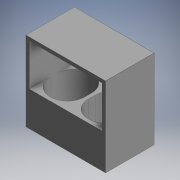
# Autodesk Inventor part: Manifold0
Saved by Autodesk Inventor 2018 (Build 220112000, 112)
## iProperties
Created: 2018-09-29
Part Number: Manifold0
Material: Generic
Document SubType Name: Modeling
Designer: Isaac Newcomb
Density: 1 g/cm^3
Appearance: Default
Author: Isaac Newcomb
Autodesk Inventor part; units mm, degrees
ref_plane "YZ Plane" through (0, 0, 0) normal (1, 0, 0) x (0, 1, 0)
ref_plane "XZ Plane" through (0, 0, 0) normal (0, 1, 0) x (-1, 0, 0)
ref_plane "XY Plane" through (0, 0, 0) normal (0, 0, 1) x (1, 0, 0)
sketch "Base Sketch" plane through (0, 0, 0) normal (0, 0, 1) x (1, 0, 0)
  line L0 (-10.5, -6) -> (10.5, -6)
  line L1 (10.5, -6) -> (10.5, 6)
  line L2 (10.5, 6) -> (-10.5, 6)
  line L3 (-10.5, 6) -> (-10.5, -6)
  line L4 (-10.5, -6) -> (10.5, 6) construction
  line L5 (10.5, -6) -> (-10.5, 6) construction
  line L6 (-11.5, 7) -> (11.5, 7)
  line L7 (11.5, 7) -> (11.5, -16)
  line L8 (11.5, -16) -> (-11.5, -16)
  line L9 (-11.5, -16) -> (-11.5, 7)
  point P0 (0, 0)
  dimension "CavityWidth" = 21
  dimension "CavityHeight" = 12
  dimension "d5" = 1
  dimension "d6" = 1
  dimension "d7" = 1
  dimension "d8" = 10
  constraints: 20 end point, 4 parallel, 2 horizontal, 2 midpoint, 2 perpendicular
  measures "CavityWidth" distance of L1.end L2.end
  measures "CavityHeight" distance of L0.end L1.end
  measures "d5" distance between parallel lines of L2 L6
  measures "d6" distance between parallel lines of L3 L9
  measures "d7" distance between parallel lines of L1 L7
  measures "d8" distance between parallel lines of L0 L8
extrude "Walls" add sketch "Base Sketch" along normal blind 14
extrude "Back" add sketch "Base Sketch" along normal blind 1 contours L3 L2 L1 L0
sketch "Whistle Hole Sketch" plane through (-10.5, -6, 14) normal (0, 1, 0) x (1, 0, 0)
  line L0 (21, 13) -> (0, 13) construction
  line L1 (0, 13) -> (0, 0) construction
  line L2 (21, 0) -> (0, 0) construction
  line L3 (21, 13) -> (21, 0) construction
  line L4 (5, 6) -> (5, 8) construction
  line L5 (10, 6) -> (10, 8)
  line L6 (0, 8) -> (0, 6)
  arc A0 (0, 6) -> (10, 6) centre (5, 6) ccw
  arc A1 (10, 8) -> (0, 8) centre (5, 8) ccw
  point P0 (10.5, 14)
  point P1 (5, 7)
  dimension "d11" = 2
  dimension "d12" = 10
  constraints: 8 end point, 5 tangent, 4 point on circle, 2 centre point, 1 collinear, 1 midpoint, 1 parallel, 1 vertical
  measures "d11" distance of L4.start L4.end
  measures "d12" diameter of A1
extrude "Whistle Hole" cut sketch "Whistle Hole Sketch" against normal up to surface (10 mm away)
pattern_linear "Rectangular Pattern2" count 2 spacing 11 along (1, 0, 0) of "Whistle Hole"
equation "\"d5\" = WallThickness"
equation "\"d6\" = WallThickness"
equation "\"d7\" = WallThickness"
equation "\"d8\" = CapLength"
equation "\"d3\" = MaxWidth + CapOvalLength + 2 * WallThickness"
equation "\"d9\" = WallThickness"
equation "\"d20\" = WallThickness"
equation "\"d30\" = MaxWidth + SpaceBtwnKeys"
equation "\"SpaceBtwnKeys\" = 1"
equation "\"WallThickness\" = 1"
equation "\"CapLength\" = 10"
equation "\"MaxWidth\" = 10"
equation "\"CapOvalLength\" = 2"
body "Solid1"
